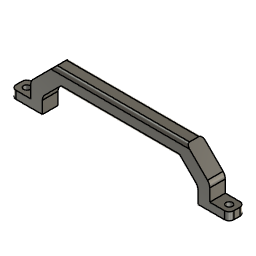
Handle v4 (Autodesk Fusion 360 design; units mm, degrees)
Autodesk Fusion 360 part; units mm, degrees
sketch "Sketch1" plane through (0, 0, 0) normal (0, 0, 1) x (1, 0, 0)
  line L0 (57.5, 5) -> (-57.5, 5)
  line L1 (-57.5, 5) -> (-57.5, -5)
  line L2 (-57.5, -5) -> (57.5, -5)
  line L3 (57.5, -5) -> (57.5, 5)
  line L4 (57.5, 5) -> (-57.5, -5) construction
  line L5 (-57.5, 5) -> (57.5, -5) construction
  line L6 (-70, -5) -> (-50, -5)
  line L7 (-50, -5) -> (-50, 5)
  line L8 (-50, 5) -> (-70, 5)
  line L9 (-70, 5) -> (-70, -5)
  line L10 (70, -5) -> (50, -5)
  line L11 (50, -5) -> (50, 5)
  line L12 (50, 5) -> (70, 5)
  line L13 (70, 5) -> (70, -5)
  dimension "d1" = 115
  dimension "d2" = 10
  dimension "d3" = 20
  dimension "d4" = 10
  dimension "d5" = 20
  dimension "d6" = 10
  constraint horizontal L0
  constraint perpendicular L0 L1
  constraint parallel L0 L2
  constraint parallel L1 L3
  constraint coincident L4 origin
  constraint coincident L5 origin
  constraint horizontal L6
  constraint vertical L7
  constraint horizontal L8
  constraint vertical L9
  constraint horizontal L10
  constraint vertical L11
  constraint horizontal L12
  constraint vertical L13
  measures "d1" distance of L1.end L2.end
  measures "d2" distance of L0.end L1.end
  measures "d3" distance of L6.start L6.end
  measures "d4" distance of L6.start L8.end
  measures "d5" distance of L10.start L10.end
  measures "d6" distance of L10.start L12.end
extrude "Extrude1" add sketch "Sketch1" along normal blind 5 contours L0 L2 L3 L10 L11 L12 | L3 L10 L12 L13 | L0 L1 L2 L6 L7 L8 | L1 L6 L8 L9 makes body 1 at (-56.6667, -1.6667, 0) makes body 2 at (56.6667, 1.6667, 0)
extrude "Extrude2" add sketch "Sketch1" along normal blind 30 contours L0 L2 L3 L10 L11 L12 | L0 L1 L2 L6 L7 L8 bodies 1 2
sketch "Sketch2" plane through (50, 0, 0) normal (-1, 0, 0) x (0, -1, 0)
  line L0 (-5, 0) -> (5, 0)
  line L1 (5, 0) -> (5, 30)
  line L2 (5, 30) -> (-5, 30)
  line L3 (-5, 30) -> (-5, 0)
  line L4 (-5, 30) -> (5, 30)
  line L5 (5, 30) -> (5, 20)
  line L6 (5, 20) -> (-5, 20)
  line L7 (-5, 20) -> (-5, 30)
  dimension "d11" = 10
  dimension "d12" = 10
  constraint horizontal L4
  constraint vertical L5
  constraint horizontal L6
  constraint vertical L7
  constraint coincident L2.end L3.start
  measures "d11" distance of L2.end L1.end
  measures "d12" distance of L2.end L6.end
extrude "Extrude3" add sketch "Sketch2" along normal blind 100 contours L1 L2 L3 L4 L5 L6 L7 bodies 1 2
chamfer "Chamfer5" distance 10 angle 45 2 edges at (50, 0, 20) (-50, 0, 20) on bodies 1
chamfer "Chamfer1" distance 15 angle 45 2 edges at (-57.5, 0, 30) (57.5, 0, 30) on bodies 1
fillet "Fillet1" radius 2 4 edges at (0, -5, 30) (0, 5, 30) (0, -5, 20) (0, 5, 20) on bodies 1
fillet "Fillet1" radius 3 4 edges at (70, -5, 2.5) (70, 5, 2.5) (-70, -5, 2.5) (-70, 5, 2.5) on bodies 1
sketch "Sketch3" plane through (0, 0, 5) normal (0, 0, 1) x (-1, 0, 0)
  arc A0 (67, -5) -> (70, -2) centre (67, -2) ccw
  line L0 (70, -2) -> (70, 2)
  arc A1 (70, 2) -> (67, 5) centre (67, 2) ccw
  line L1 (67, 5) -> (57.5, 5)
  line L2 (57.5, -5) -> (67, -5)
  circle A2 centre (65, 0) radius 2.1
  line L3 (57.5, 5) -> (57.5, -5)
  dimension "d24" = 4.2
  measures "d24" diameter of A2
sketch "Sketch4" plane through (0, 0, 5) normal (0, 0, 1) x (-1, 0, 0)
  arc A0 (-70, -2) -> (-67, -5) centre (-67, -2) ccw
  line L0 (-67, -5) -> (-57.5, -5)
  line L1 (-57.5, 5) -> (-67, 5)
  arc A1 (-67, 5) -> (-70, 2) centre (-67, 2) ccw
  line L2 (-70, 2) -> (-70, -2)
  circle A2 centre (-65, 0) radius 2.1
  line L3 (-57.5, -5) -> (-57.5, 5)
  dimension "d25" = 4.2
  measures "d25" diameter of A2
extrude "Extrude4" cut sketch "Sketch4" sketch "Sketch3" against normal blind 5 contours A2 of sketch 2 contours A2 bodies 1
sketch "Sketch5" plane through (0, 0, 5) normal (0, 0, 1) x (-1, 0, 0)
  circle A0 centre (65, 0) radius 2.1
  arc A1 (67, -5) -> (70, -2) centre (67, -2) ccw
  line L0 (70, -2) -> (70, 2)
  arc A2 (70, 2) -> (67, 5) centre (67, 2) ccw
  line L1 (67, 5) -> (57.5, 5)
  line L2 (57.5, -5) -> (67, -5)
  circle A3 centre (65, 0) radius 3.5
  line L3 (57.5, 5) -> (57.5, -5)
  dimension "d28" = 7
  constraint concentric A0 A3
  measures "d28" diameter of A3
fillet "Fillet2" radius 5 4 edges at (50, 0, 10) (-50, 0, 10) (57.5, 0, 15) (-57.5, 0, 15) on bodies 1
